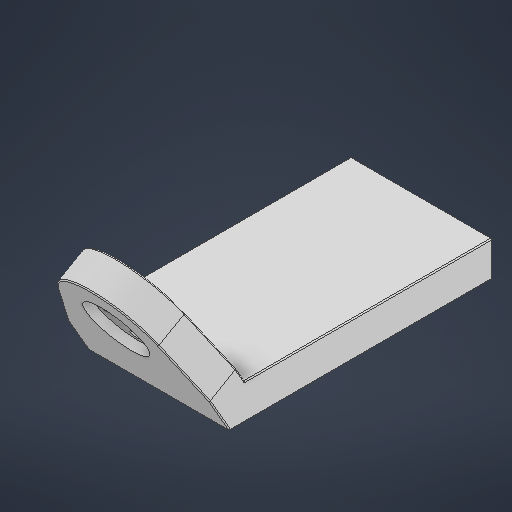
# Autodesk Inventor part: rearTorso30Deg
Saved by Autodesk Inventor 2026 (Build 300175000, 175)
## iProperties
Created: 2025-05-29
Part Number: rearTorso30Deg
Material: Generic
Document SubType Name: Modeling
Designer: Elizabeth
Density: 1 g/cm^3
Appearance: Default
Author: Elizabeth
Autodesk Inventor part; units mm, degrees
ref_plane "YZ Plane" through (0, 0, 0) normal (1, 0, 0) x (0, 1, 0)
ref_plane "XZ Plane" through (0, 0, 0) normal (0, 1, 0) x (-1, 0, 0)
sketch "Sketch1" plane through (0, 0, 0) normal (1, 0, 0) x (0, 1, 0)
  line L0 (0, -80) -> (10, -80)
  line L1 (10, -80) -> (10, -10)
  line L2 (10, -10) -> (41.9301, -10)
  line L3 (10, -10) -> (41.9301, 8.4349)
  line L4 (10, -10) -> (36.6272, -10) construction
  line L5 (37.6, 15.9349) -> (0, -5.7735)
  line L6 (37.6, 15.9349) -> (0, 15.9349)
  line L7 (0, 15.9349) -> (0, -80)
  line L8 (37.6, 15.9349) -> (41.9301, 8.4349)
  line L9 (41.9301, 8.4349) -> (41.9301, -10)
  point P0 (0, 0)
  dimension "d4" = 30
  constraints: 20 end point, 2 horizontal, 2 vertical, 1 parallel, 1 perpendicular
  measures "d4" angle of L4 L3
extrude "Extrusion1" add sketch "Sketch1" against normal blind 40 contours L7 L5 L8 L3 L1 L0
ref_plane "Work Plane3" through (-40, 0, -5.7735) normal (0, -0.5, 0.866) x (1, 0, 0)
sketch "Sketch3" plane through (-40, 0, -5.7735) normal (0, -0.5, 0.866) x (1, 0, 0)
  line L0 (40, 45.0131) -> (0, 45.0131)
  line L1 (0, 11.5378) -> (40, 11.5378)
  line L2 (0, 11.5378) -> (0, 45.0131)
  line L3 (40, 45.0131) -> (40, 11.5378)
  circle A0 centre (20, 24.1378) radius 15
  circle A1 centre (20, 24.1378) radius 8.5
  line L4 (0, 11.5378) -> (0, 45.0131)
  line L5 (0, 11.5378) -> (5.7669, 28.8728)
  line L6 (40, 11.5378) -> (34.2331, 28.8728)
  circle A2 centre (20, 24.1378) radius 6
  circle A3 centre (20, 30.1378) radius 1.2
  circle A4 centre (26, 24.1378) radius 1.2
  circle A5 centre (20, 18.1378) radius 1.2
  circle A6 centre (14, 24.1378) radius 1.2
  point P0 (40, 2.8868)
  point P1 (20, 39.4287)
  point P2 (11.8612, 11.5378)
  point P3 (28.1388, 11.5378)
  dimension "d19" = 30
  dimension "d20" = 17
  dimension "d21" = 12
  dimension "d22" = 2.4
  dimension "d23" = 2.4
  dimension "d24" = 2.4
  dimension "d25" = 2.4
  constraints: 14 end point, 7 centre point, 6 point on circle, 2 coincident, 2 tangent, 1 parallel, 1 perpendicular
  measures "d19" diameter of A0
  measures "d20" diameter of A1
  measures "d21" diameter of A2
  measures "d22" diameter of A3
  measures "d23" diameter of A4
  measures "d24" diameter of A5
  measures "d25" diameter of A6
extrude "Extrusion4" cut sketch "Sketch3" against normal up to surface (8.6603 mm away) contours L3 L6 A0 L5 L2 L0 | A2 A4 | A2 A4 | A3 A2 | A2 A3 | A5 A2 | A2 A5 | A6 A2 | A2 A6
extrude "Extrusion5" cut sketch "Sketch3" against normal blind 2.5 contours A1 | A2 A4 | A2 A4 | A4 A2 A5 A6 A3 | A3 A2 | A2 A3 | A5 A2 | A2 A5 | A6 A2 | A2 A6
sketch "Sketch5" plane through (0, 10, -10) normal (0, 0.5, -0.866) x (-1, 0, 0)
  circle A0 centre (20, 23.5908) radius 1.2 projected
  circle A1 centre (20, 23.5908) radius 2.5
  circle A2 centre (14, 17.5908) radius 1.2 projected
  circle A3 centre (14, 17.5908) radius 2.5
  circle A4 centre (26, 17.5908) radius 1.2 projected
  circle A5 centre (26, 17.5908) radius 2.5
  circle A6 centre (20, 11.5908) radius 1.2 projected
  circle A7 centre (20, 11.5908) radius 2.5
  point P0 (0, -3.6603)
  dimension "d30" = 5
  dimension "d31" = 5
  dimension "d32" = 5
  dimension "d33" = 5
  constraints: 4 centre point, 4 coincident
  measures "d30" diameter of A1
  measures "d31" diameter of A3
  measures "d32" diameter of A5
  measures "d33" diameter of A7
extrude "Extrusion6" cut sketch "Sketch5" against normal blind 2 contours A0 | A1 | A2 | A3 | A4 | A5 | A6 | A7
fillet "Fillet1" radius 0.3 19 edges at (-40, 10, -45) (-40, 12.1611, -8.7523) (-20, 33.8943, 13.7954) (-2.8835, 17.4983, 4.3291) (-37.1165, 17.4983, 4.3291) (-20, 38.2244, 6.2954) (-2.8835, 21.8284, -3.1709) (-37.1165, 21.8284, -3.1709) (-40, 4.996, -2.8891) (-20, 10, -80) (-40, 5, -80) (-40, 0, -42.8868) (-20, 0, -5.7735) (-20, 0, -80) (0, 5, -80) (0, 10, -45) (0, 4.996, -2.8891) (0, 0, -42.8868) (0, 12.1611, -8.7523)
body "Solid1"
